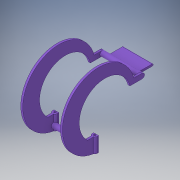
# Autodesk Inventor part: Mouth-Upper-Lip
Saved by Autodesk Inventor 2018.3 (Build 223284000, 284)
## iProperties
Created: 2018-05-17
Part Number: Mouth-Upper-Lip
Material: Generisch
Document SubType Name: Modeling
Designer: JochenAlt
Density: 1 g/cm^3
Appearance: Violett
Author: JochenAlt
Autodesk Inventor part; units mm, degrees
ref_plane "XZ Plane" through (0, 0, 0) normal (0, 1, 0) x (-1, 0, 0)
ref_plane "XY Plane" through (0, 0, 0) normal (0, 0, 1) x (1, 0, 0)
sketch "Skizze4" plane through (0, 0, 0) normal (0, 0, 1) x (1, 0, 0)
  line L0 (0, 2.3) -> (0, -3.3) construction
  line L1 (-31.5, 0) -> (31.5, 0) construction
  arc A0 (-22.5, 0) -> (-17.5, 0) centre (-20, 0) ccw
  arc A1 (17.5, 0) -> (22.5, 0) centre (20, 0) ccw
  circle A2 centre (-20, 0) radius 1
  circle A3 centre (20, 0) radius 1
  line L2 (-22.5, 0) -> (-22.5, 1.5)
  line L3 (-22.5, 1.5) -> (-17.5, 1.5)
  line L4 (-17.5, 1.5) -> (-17.5, 0)
  line L5 (17.5, 0) -> (17.5, 1.5)
  line L6 (17.5, 1.5) -> (22.5, 1.5)
  line L7 (22.5, 1.5) -> (22.5, 0)
  point P0 (0, 0)
  dimension "d24" = 40
  dimension "d25" = 2
  dimension "d26" = 5
  dimension "d27" = 1.5
  constraints: 12 end point, 4 centre point, 4 point on circle, 2 coincident, 2 equal radius, 2 perpendicular, 2 tangent, 2 vertical, 1 collinear, 1 symmetric about line, 7 other
  measures "d24" distance of A1.centre A0.centre
  measures "d25" diameter of A2
  measures "d26" diameter of A0
  measures "d27" distance from line of L3 A0.centre
extrude "Extrusion6" add sketch "Skizze4" along normal blind 14.8
sketch "Skizze6" plane through (0, 0, 0) normal (1, 0, 0) x (0, 1, 0)
  line L0 (-1, 0) -> (-1, 14.8) projected
  line L1 (-8.1796, 14.8) -> (-1, 14.8)
  line L2 (-1, 14.8) -> (-1, 0)
  arc A0 (38.5248, 45.8548) -> (-2.5, 0) centre (3.1485, 36.2257) ccw
  line L3 (-1, 0) -> (-2.5, 0)
  line L4 (0, 0) -> (-2.5, 0) projected
  line L5 (0, 14.8) -> (-2.5, 14.8) construction
  line L6 (1.5, 0) -> (1.5, 14.8) construction
  line L7 (1.5, 14.8) -> (0, 14.8) construction
  circle A1 centre (9.5, 34) radius 24.1 construction
  arc A2 (34.6838, 40.8548) -> (-8.1796, 14.8) centre (9.5, 34) ccw
  line L8 (38.5248, 45.8548) -> (38.4377, 46.1749) construction
  line L9 (34.6838, 40.8548) -> (34.9556, 39.8562) construction
  line L10 (34.6838, 40.8548) -> (46.8107, 40.8548)
  line L11 (38.5248, 45.8548) -> (46.8107, 45.8548)
  circle A3 centre (-2.0969, 5.0692) radius 2.5
  line L12 (-2.5119, 2.6039) -> (-2.9383, 0.0711) construction
  line L13 (-1.1667, 7.3898) -> (-0.211, 9.7739) construction
  line L14 (63.1485, 42.8548) -> (49.2601, 42.8548)
  line L15 (46.8107, 40.8548) -> (63.1485, 40.8548)
  circle A4 centre (46.8107, 43.3548) radius 2.5
  arc A5 (63.1485, 40.8548) -> (63.1485, 42.8548) centre (63.1485, 41.8548) ccw
  dimension "d44" = 8
  dimension "d45" = 19.2
  dimension "d47" = 48.2
  dimension "d48" = 2
  dimension "d58" = 5
  dimension "d59" = 1.9999
  dimension "d62" = 60
  constraints: 22 end point, 13 point on circle, 6 centre point, 6 tangent, 4 horizontal, 4 line through centre, 3 point on line, 2 parallel, 2 perpendicular, 1 coincident, 1 concentric, 1 equal length, 1 equal radius
  measures "d44" distance from line of L6 point (9.5, 34)
  measures "d45" distance from line of L7 point (9.5, 34)
  measures "d47" diameter of A1
  measures "d48" radial gap between concentric circles of A2 A1
  measures "d58" diameter of A4
  measures "d59" distance between parallel lines of L15 L14
  measures "d62" horizontal distance of A0.centre A5.centre
ref_plane "Arbeitsebene3" through (20, 0, 0) normal (1, 0, 0) x (0, 1, 0)
ref_plane "Arbeitsebene4" through (-20, 0, 0) normal (1, 0, 0) x (0, 1, 0)
extrude "Extrusion8" add sketch "Skizze6" along normal mid plane 2 from surface at 20 contours L3 A0 L11 A4 L10 A2 L1 L0 A3 | A3 L0 | A4 picked at (-2.1463, 5.3607)
extrude "Extrusion9" add sketch "Skizze6" along normal mid plane 2 from surface at -20 contours L3 A0 L11 A4 L10 A2 L1 L0 A3 | A3 L0 | A4 picked at (-2.1463, 5.3607)
extrude "Extrusion10" add sketch "Skizze6" against normal up to surface (38 mm away) from surface at 19 contours A3 L0 | L0 A3 | A4
extrude "Extrusion11" add sketch "Skizze6" along normal mid plane 30 contours A4 L14 A5 L15
